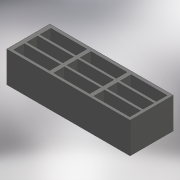
# Autodesk Inventor part: 1420-14-06 Meuble noir
Saved by Autodesk Inventor 2017 (Build 210142000, 142)
## iProperties
Company: FABLAB Frenchmakers
Part Number: 1420-14-06 Meuble noir
Project: 1420 VAUBAN 3D XL
Material: Bois (bouleau)
Catalog Web Link: http://www.frenchmakers.com/
Document SubType Name: Modeling
Designer: Adrien MARY
Mass: 132344 g
Surface Area: 104875 cm^2
Volume: 240625 cm^3
Density: 0.55 g/cm^3
Appearance: Lisse - Noir(1)
Author: Adrien MARY
Autodesk Inventor part; units mm, degrees
ref_plane "YZ Plane" through (0, 0, 0) normal (1, 0, 0) x (0, 1, 0)
ref_plane "XZ Plane" through (0, 0, 0) normal (0, 1, 0) x (-1, 0, 0)
ref_plane "XY Plane" through (0, 0, 0) normal (0, 0, 1) x (1, 0, 0)
sketch "Esquisse1" plane through (0, 0, 0) normal (0, 0, 1) x (1, 0, 0)
  line L0 (-1000, -350) -> (1000, -350)
  line L1 (1000, -350) -> (1000, 350)
  line L2 (1000, 350) -> (-1000, 350)
  line L3 (-1000, 350) -> (-1000, -350)
  line L4 (-1000, -350) -> (1000, 350) construction
  line L5 (1000, -350) -> (-1000, 350) construction
  point P0 (0, 0)
  dimension "d0" = 2000
  dimension "d1" = 700
  constraints: 12 end point, 2 midpoint, 2 parallel, 1 horizontal, 1 perpendicular
  measures "d0" distance of L2.end L1.end
  measures "d1" distance of L1.end L0.end
extrude "Extrusion1" add sketch "Esquisse1" along normal blind 500
sketch "Esquisse3" plane through (0, 0, 0) normal (0, 0, -1) x (-1, 0, 0)
  line L0 (-950, 125) -> (-366.6667, 125)
  line L1 (-366.6667, 125) -> (-366.6667, 300)
  line L2 (-366.6667, 300) -> (-950, 300)
  line L3 (-950, 300) -> (-950, 125)
  line L4 (-1000, 350) -> (1000, 350) projected
  line L5 (-1000, -350) -> (-1000, 350) projected
  point P0 (0, 0)
  dimension "d4" = 175
  dimension "d5" = 583.3333
  dimension "d6" = 50
  dimension "d7" = 50
  constraints: 8 end point, 2 parallel, 1 horizontal, 1 perpendicular
  measures "d4" distance of L2.end L0.start
  measures "d5" distance of L1.end L2.end
  measures "d6" distance between parallel lines of L4 L2
  measures "d7" distance between parallel lines of L5 L3
extrude "Extrusion2" cut sketch "Esquisse3" against normal through all
pattern_linear "Réseau rectangulaire1" count 3 spacing 650 along (-1, 0, 0) of "Extrusion2"
pattern_linear "Réseau rectangulaire2" count 3 spacing 215 along (0, -1, 0) of "Extrusion2", "Réseau rectangulaire1"
